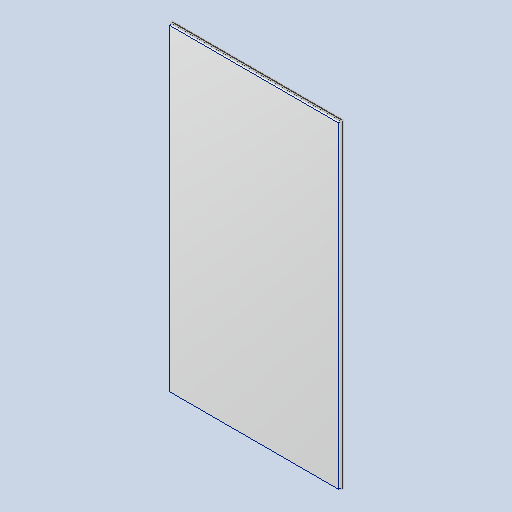
# Autodesk Inventor part: field
Saved by Autodesk Inventor 2025.2 (Build 292293000, 293)
## iProperties
Created: 2024-12-29
Part Number: field
Material: アルミニウム 6061
Document SubType Name: Modeling
Designer: haruy
Density: 2.7 g/cm^3
Appearance: アルミニウム - フラット
Author: haruy
Autodesk Inventor part; units mm, degrees
ref_plane "YZ Plane" through (0, 0, 0) normal (1, 0, 0) x (0, 1, 0)
ref_plane "XZ Plane" through (0, 0, 0) normal (0, 1, 0) x (-1, 0, 0)
ref_plane "XY Plane" through (0, 0, 0) normal (0, 0, 1) x (1, 0, 0)
sketch "スケッチ2" plane through (0, 0, 0) normal (0, 0, 1) x (1, 0, 0)
  line L0 (4000, -7500) -> (-4000, -7500)
  line L1 (-4000, -7500) -> (-4000, 7500)
  line L2 (-4000, 7500) -> (4000, 7500)
  line L3 (4000, 7500) -> (4000, -7500)
  line L4 (4000, -7500) -> (-4000, 7500) construction
  line L5 (-4000, -7500) -> (4000, 7500) construction
  line L6 (4050, 7550) -> (-4050, 7550)
  line L7 (-4050, 7550) -> (-4050, -7550)
  line L8 (-4050, -7550) -> (4050, -7550)
  line L9 (4050, -7550) -> (4050, 7550)
  point P0 (0, 0)
  dimension "d0" = 8000
  dimension "d1" = 15000
  dimension "d2" = 50
  constraints: 20 end point, 4 parallel, 2 midpoint, 2 perpendicular, 1 horizontal, 3 other
  measures "d0" distance of L1.end L2.end
  measures "d1" distance of L0.end L1.end
  measures "d2" distance between parallel lines of L2 L6
extrude "押し出し1" add sketch "スケッチ2" along normal blind 100 contours L0 L1 L2 L3
extrude "押し出し2" add sketch "スケッチ2" against normal blind 100 separate body
